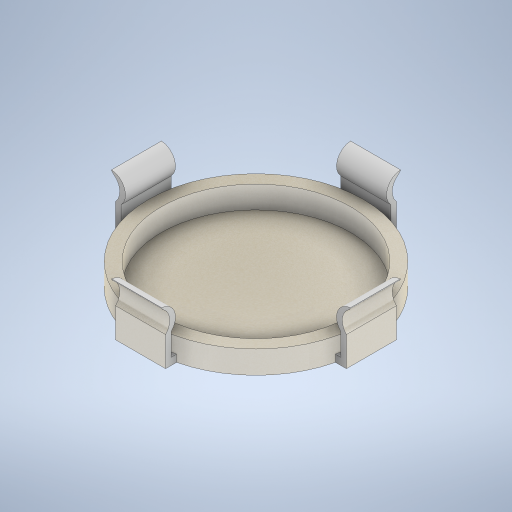
# Autodesk Inventor part: TapaContenedorTest
Saved by Autodesk Inventor 2024 (Build 280153000, 153)
## iProperties
Created: 2024-05-15
Part Number: TapaContenedorTest
Material: Genérico
Document SubType Name: Modeling
Designer: alexa
Density: 1 g/cm^3
Appearance: Valor por defecto
Author: alexa
Autodesk Inventor part; units mm, degrees
ref_plane "YZ Plane" through (0, 0, 0) normal (1, 0, 0) x (0, 1, 0)
ref_plane "XZ Plane" through (0, 0, 0) normal (0, 1, 0) x (-1, 0, 0)
ref_plane "XY Plane" through (0, 0, 0) normal (0, 0, 1) x (1, 0, 0)
sketch "Sketch1" plane through (0, 0, 0) normal (0, 1, 0) x (-1, 0, 0)
  circle A0 centre (0, 0) radius 50.9
  dimension "d0" = 101.8
  constraints: 1 centre point, 1 coincident
  measures "d0" diameter of A0
extrude "Extrusion1" add sketch "Sketch1" along normal blind 0.2
sketch "Sketch2" plane through (0, 0.2, 0) normal (0, 1, 0) x (1, 0, 0)
  circle A0 centre (0, 0) radius 50.9
  circle A1 centre (0, 0) radius 44.9
  dimension "d3" = 6
  constraints: 2 centre point, 1 coincident
  measures "d3" radial gap between concentric circles of A0 A1
extrude "Extrusion2" add sketch "Sketch2" along normal blind 10.6
sketch "Sketch3" plane through (0, 0, 0) normal (0, -1, 0) x (1, 0, 0)
  circle A0 centre (0, 0) radius 50.9 projected
  line L0 (-54.7, -11.85) -> (-54.7, 11.85)
  line L1 (-54.7, -11.85) -> (-49.5014, -11.85)
  line L2 (-54.7, 11.85) -> (-49.5014, 11.85)
  dimension "d8" = 23.7
  constraints: 6 end point, 2 point on circle, 1 horizontal, 1 parallel
  measures "d8" distance of L0.start L0.end
extrude "Extrusion3" add sketch "Sketch3" against normal blind 3.4 contours A0 L1 L0 L2
sketch "Sketch4" plane through (0, 3.4, 0) normal (0, 1, 0) x (1, 0, 0)
  line L0 (-54.7, 11.85) -> (-54.7, -11.85) projected
  line L1 (-54.7, -11.85) -> (-52, -11.85)
  line L2 (-52, -11.85) -> (-52, 11.85)
  line L3 (-52, 11.85) -> (-54.7, 11.85)
  line L4 (-54.7, 11.85) -> (-54.7, -11.85)
  point P0 (0, 0)
  dimension "d11" = 2.7
  constraints: 8 end point, 2 parallel, 1 horizontal, 1 perpendicular
  measures "d11" distance of L3.end L2.end
extrude "Extrusion4" add sketch "Sketch4" along normal blind 10.6
sketch "Sketch6" plane through (-54.7, 0, 11.85) normal (0, 0, 1) x (1, 0, 0)
  line L0 (2.7, 14) -> (0, 14) projected
  line L1 (-1.9318, 26) -> (-2.8707, 26)
  arc A0 (2.7, 14) -> (-2.8707, 26) centre (-2.4013, 18.9249) ccw
  arc A1 (0, 14) -> (-5.5707, 26) centre (-5.1013, 18.9249) ccw
  line L2 (-2.8707, 26) -> (-5.5707, 26)
  point P0 (54.7, 0)
  point P1 (-4.6318, 26)
  point P2 (-4.6318, 26)
  dimension "d15" = 2.7
  dimension "d18" = 2.7
  constraints: 6 point on circle, 4 end point, 3 horizontal, 2 centre point, 5 other
  measures "d15" distance of L0.start L0.end
  measures "d18" distance of A0.centre A1.centre
extrude "Extrusion5" add sketch "Sketch6" against normal blind 23.7 contours L0 A1 L2 L1 A0
fillet "Fillet1" radius 2 1 edges at (-59.3318, 26, 0)
pattern_circular "Circular Pattern1" count 4 over 360 about axis through (0, -10, 0) along (0, 1, 0) of "Fillet1", "Extrusion5", "Extrusion4", "Extrusion3"
body "Solid1"
